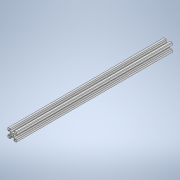
# Autodesk Inventor part: Профиль_аллюминиевый355
Saved by Autodesk Inventor 2020 (Build 240168000, 168)
## iProperties
Created: 2019-09-17
Part Number: Профиль_аллюминиевый355
Material: Типовые
Document SubType Name: Modeling
Designer: Михаил
Density: 1 g/cm^3
Appearance: По умолчанию
Author: Михаил
Autodesk Inventor part; units mm, degrees
ref_plane "YZ Plane" through (0, 0, 0) normal (1, 0, 0) x (0, 1, 0)
ref_plane "XZ Plane" through (0, 0, 0) normal (0, 1, 0) x (-1, 0, 0)
ref_plane "XY Plane" through (0, 0, 0) normal (0, 0, 1) x (1, 0, 0)
sketch "Эскиз1" plane through (0, 0, 0) normal (0, 0, 1) x (1, 0, 0)
  line L0 (-4.8, 10) -> (-3, 8.2)
  line L1 (-4.8, 10) -> (-2.2544, 10) construction
  line L2 (4.8, 10) -> (3, 8.2)
  line L3 (4.8, 10) -> (7.3456, 10) construction
  line L4 (10, 4.8) -> (8.2, 3)
  arc A0 (-9, 10) -> (-10, 9) centre (-9, 9) ccw
  arc A1 (10, 9) -> (9, 10) centre (9, 9) ccw
  arc A2 (-10, -9) -> (-9, -10) centre (-9, -9) ccw
  arc A3 (8.9996, -10) -> (10, -9) centre (9, -9) ccw
  line L5 (0, 3.9) -> (-2.7, 3.9)
  line L6 (0, 3.9) -> (2.7, 3.9)
  line L7 (3, 8.2) -> (5.5, 8.2)
  line L8 (2.7, 3.9) -> (5.5, 6.7)
  line L9 (5.5, 6.7) -> (5.5, 8.2)
  line L10 (3.9, 0) -> (3.9, 2.7)
  line L11 (3.9, 0) -> (3.9, -2.7)
  line L12 (3.9, 2.7) -> (6.7, 5.5)
  line L13 (3.9, 2.7) -> (7.8598, 2.7) construction
  line L14 (9, 10) -> (4.8, 10)
  line L15 (-4.8, 10) -> (-9, 10)
  line L16 (0, -3.9) -> (-2.7, -3.9)
  line L17 (0, -3.9) -> (2.7, -3.9)
  line L18 (-3.9, 0) -> (-3.9, -2.7)
  line L19 (-3.9, 0) -> (-3.9, 2.7)
  line L20 (8.2, 3) -> (8.2, 5.5)
  line L21 (8.2, 5.5) -> (6.7, 5.5)
  line L22 (-10, -4.8) -> (-7.4544, -4.8) construction
  line L23 (-4.8, -10) -> (-3, -8.2)
  line L24 (-4.8, -10) -> (-2.2544, -10) construction
  line L25 (4.7996, -10) -> (2.9996, -8.2)
  line L26 (4.7996, -10) -> (7.3452, -10) construction
  line L27 (10, -4.8) -> (8.2, -3)
  line L28 (8.9996, -10) -> (4.7996, -10)
  line L29 (-9, -10) -> (-4.8, -10)
  line L30 (10, -4.8) -> (10, -9)
  line L31 (10, 9) -> (10, 4.8)
  line L32 (-10, -4.8) -> (-10, -9)
  line L33 (-3, 8.2) -> (-5.5, 8.2)
  line L34 (-2.7, 3.9) -> (-5.5, 6.7)
  line L35 (-2.7, 3.9) -> (1.2598, 3.9) construction
  line L36 (-5.5, 6.7) -> (-5.5, 8.2)
  line L37 (-3.9, 2.7) -> (-6.7, 5.5)
  line L38 (-6.7, 5.5) -> (-8.2, 5.5)
  line L39 (-8.2, -3) -> (-8.2, -5.5)
  line L40 (-3, -8.2) -> (-5.5, -8.2)
  line L41 (2.9996, -8.2) -> (5.5, -8.2)
  line L42 (8.2, -3) -> (8.2, -5.5)
  line L43 (-3.9, -2.7) -> (-6.7, -5.5)
  line L44 (-6.7, -5.5) -> (-8.2, -5.5)
  line L45 (-2.7, -3.9) -> (-5.5, -6.7)
  line L46 (-5.5, -6.7) -> (-5.5, -8.2)
  line L47 (-10, 9) -> (-10, 4.8)
  line L48 (-10, 4.8) -> (-8.2, 3)
  line L49 (-8.2, 5.5) -> (-8.2, 3)
  line L50 (-10, -4.8) -> (-8.2, -3)
  line L51 (2.7, -3.9) -> (5.5, -6.7)
  line L52 (5.5, -6.7) -> (5.5, -8.2)
  line L53 (3.9, -2.7) -> (6.7, -5.5)
  line L54 (6.7, -5.5) -> (8.2, -5.5)
  point P0 (0, 0)
  dimension "d16" = 45
  dimension "d17" = 135
  dimension "d25" = 6
  dimension "d29" = 1
  dimension "d30" = 1
  dimension "d31" = 2.7
  dimension "d32" = 2.7
  dimension "d34" = 2.5
  dimension "d36" = 2.7
  dimension "d37" = 2.7
  dimension "d38" = 3.9
  dimension "d39" = 45
  dimension "d42" = 2.7
  dimension "d43" = 2.7
  dimension "d44" = 3.9
  dimension "d45" = 2.7
  dimension "d46" = 2.7
  dimension "d48" = 10
  dimension "d49" = 10
  dimension "d55" = 4.5
  dimension "d58" = 9
  dimension "d59" = 9
  dimension "d60" = 2.5
  dimension "d61" = 2.8
  dimension "d63" = 1.6971
  dimension "d65" = 45
  dimension "d67" = 135
  dimension "d73" = 10
  dimension "d74" = 10
  dimension "d77" = 18
  dimension "d78" = 18
  dimension "d79" = 135
  dimension "d80" = 135
  dimension "d81" = 4.5
  dimension "d82" = 1.8
  dimension "d83" = 1.8
  dimension "d84" = 1
  dimension "d85" = 1
  dimension "d87" = 4.5
  dimension "d89" = 1.8
  dimension "d91" = 135
  dimension "d92" = 1.6971
  dimension "d94" = 4.5
  dimension "d95" = 1.8
  dimension "d96" = 4.5
  dimension "d97" = 1.8
  dimension "d98" = 4.5
  dimension "d99" = 1.8
  dimension "d100" = 1.8
  dimension "d107" = 4.2
  dimension "d108" = 10
  dimension "d109" = 4.5
  dimension "d110" = 1.8
  dimension "d111" = 135
  dimension "d112" = 4.2
  dimension "d113" = 4.2
  dimension "d114" = 6
  dimension "d115" = 135
  dimension "d116" = 1.6971
  dimension "d117" = 4.2
  dimension "d118" = 4.2
  dimension "d119" = 4.5
  dimension "d120" = 135
  dimension "d121" = 1.5
  constraints: 110 end point, 20 horizontal, 14 vertical, 10 equal length, 8 point on circle, 4 centre point, 2 equal radius, 2 perpendicular, 2 point on line
  measures "d16" angle of L0 L1
  measures "d17" angle of L2 L3
  measures "d25" distance of L2.end L0.end
  measures "d29" radius of A0
  measures "d30" radius of A1
  measures "d31" distance of L5.start L5.end
  measures "d32" distance of L5.start L6.end
  measures "d34" distance of L2.end L7.end
  measures "d36" distance of L10.start L10.end
  measures "d37" distance of L10.start L11.end
  measures "d38" distance from line of L10 point (0, 0)
  measures "d39" angle of L13 L12
  measures "d42" distance of L16.start L16.end
  measures "d43" distance of L16.start L17.end
  measures "d44" distance from line of L16 point (0, 0)
  measures "d45" distance of L18.start L18.end
  measures "d46" distance of L18.start L19.end
  measures "d48" distance from line of L14 point (0, 0)
  measures "d49" distance from line of L15 point (0, 0)
  measures "d55" distance from line of L20.end L14
  measures "d58" horizontal distance of point (0, 0) A2.centre
  measures "d59" horizontal distance of point (0, 0) A1.centre
  measures "d60" distance of L4.end L20.end
  measures "d61" horizontal distance of L10.end L12.end
  measures "d63" distance between parallel lines of L8 L12
  measures "d65" angle of L24 L23
  measures "d67" angle of L26 L25
  measures "d73" distance from line of L32 point (0, 0)
  measures "d74" distance from line of L29 point (0, 0)
  measures "d77" distance of A1.centre A0.centre
  measures "d78" distance of A3.centre A1.centre
  measures "d79" angle of L4 L31
  measures "d80" angle of L27 L30
  measures "d81" distance between parallel lines of L9 L31
  measures "d82" distance between parallel lines of L20 L31
  measures "d83" distance between parallel lines of L7 L3
  measures "d84" distance from line of A2.centre L32
  measures "d85" distance from line of A3.centre L30
  measures "d87" distance from line of L38.end L15
  measures "d89" distance between parallel lines of L33 L15
  measures "d91" angle of L35 L34
  measures "d92" distance between parallel lines of L37 L34
  measures "d94" distance from line of L39.end L29
  measures "d95" distance between parallel lines of L39 L32
  measures "d96" distance from line of L40.end L32
  measures "d97" distance between parallel lines of L40 L29
  measures "d98" distance from line of L41.end L30
  measures "d99" distance between parallel lines of L42 L30
  measures "d100" distance between parallel lines of L41 L28
  measures "d107" distance of L47.start L47.end
  measures "d108" distance from line of L47 point (0, 0)
  measures "d109" distance between parallel lines of L36 L47
  measures "d110" distance between parallel lines of L49 L47
  measures "d111" angle of L48 L47
  measures "d112" distance of L22.start L32.end
  measures "d113" distance of L29.start L23.start
  measures "d114" distance of L39.start L49.end
  measures "d115" angle of L43 L44
  measures "d116" distance between parallel lines of L45 L43
  measures "d117" distance of L25.start L28.start
  measures "d118" distance of L27.start L30.end
  measures "d119" distance from line of L42.end L28
  measures "d120" angle of L53 L11
  measures "d121" distance of L53.end L54.end
extrude "Выдавливание2" add sketch "Эскиз1" along normal blind 355
sketch "Эскиз2" plane through (0, 0, 355) normal (0, 0, 1) x (1, 0, 0)
  circle A0 centre (0, 0) radius 2.1
  dimension "d131" = 4.2
  constraints: 1 centre point, 1 coincident
  measures "d131" diameter of A0
extrude "Выдавливание3" cut sketch "Эскиз2" against normal through all
